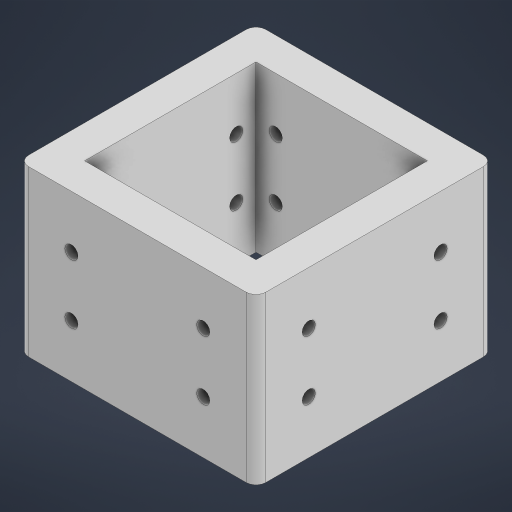
# Autodesk Inventor part: centerlegg_mounting_bracket
Saved by Autodesk Inventor 2024 (Build 280153000, 153)
## iProperties
Created: 2023-05-23
Part Number: centerlegg_mounting_bracket
Material: Generic
Document SubType Name: Modeling
Designer: aasmu
Density: 1 g/cm^3
Appearance: Default
screw_size: 4.000 mm
boarder_to_hole: 16.000 mm
bracket_height: 50.000 mm
Author: aasmu
Autodesk Inventor part; units mm, degrees
ref_plane "YZ Plane" through (0, 0, 0) normal (1, 0, 0) x (0, 1, 0)
ref_plane "XZ Plane" through (0, 0, 0) normal (0, 1, 0) x (-1, 0, 0)
ref_plane "XY Plane" through (0, 0, 0) normal (0, 0, 1) x (1, 0, 0)
sketch "Sketch1" plane through (0, 0, 0) normal (0, 1, 0) x (-1, 0, 0)
  line L0 (0, 0) -> (72, 0)
  line L1 (72, 0) -> (72, -72)
  line L2 (72, -72) -> (0, -72)
  line L3 (0, -72) -> (0, 0)
  line L4 (62, -10) -> (10, -10)
  line L5 (10, -10) -> (10, -62)
  line L6 (10, -62) -> (62, -62)
  line L7 (62, -62) -> (62, -10)
  line L8 (36, 0) -> (36, -10) construction
  line L9 (10, -36) -> (0, -36) construction
  dimension "d1" = 52
  dimension "d3" = 10
  constraints: 20 end point, 4 midpoint, 4 parallel, 4 perpendicular, 3 horizontal, 1 vertical
  measures "d1" distance of L5.end L6.end
  measures "d3" distance between parallel lines of L7 L1
extrude "Extrusion1" add sketch "Sketch1" along normal blind 50
sketch "Sketch2" plane through (-72, 0, 0) normal (0, 0, 1) x (1, 0, 0)
  line L0 (10, 50) -> (62, 50) construction
  line L1 (16, 50) -> (16, 34) construction
  line L2 (16, 16) -> (16, 0) construction
  line L3 (16, 34) -> (0, 34) construction
  line L4 (0, 0) -> (0, 50) construction
  line L5 (56, 50) -> (56, 34) construction
  line L6 (56, 34) -> (72, 34) construction
  line L7 (72, 0) -> (72, 50) construction
  line L8 (72, 16) -> (56, 16) construction
  line L9 (56, 16) -> (56, 0) construction
  circle A0 centre (16, 34) radius 2
  circle A1 centre (56, 34) radius 2
  circle A2 centre (56, 16) radius 2
  circle A3 centre (16, 16) radius 2
  line L10 (0, 0) -> (72, 0) construction
  dimension "boarder_to_hole" = 16
  dimension "d7" = 4
  constraints: 15 end point, 7 point on line, 6 equal length, 4 centre point, 4 coincident, 3 equal radius, 2 horizontal, 2 perpendicular, 2 vertical, 1 collinear
  measures "boarder_to_hole" distance of L1.end L1.start
  measures "d7" diameter of A0
extrude "Extrusion2" cut sketch "Sketch2" against normal up to surface (72 mm away)
sketch "Sketch3" plane through (0, 0, 0) normal (1, 0, 0) x (0, 0, -1)
  line L0 (0, 50) -> (60.8888, 50) construction
  line L1 (16, 50) -> (16, 34) construction
  line L2 (16, 16) -> (16, 0) construction
  line L3 (16, 34) -> (0, 34) construction
  line L4 (0, 0) -> (0, 50) construction
  line L5 (56, 50) -> (56, 34) construction
  line L6 (56, 34) -> (72, 34) construction
  line L7 (72, 0) -> (72, 49.9084) construction
  line L8 (72, 16) -> (56, 16) construction
  line L9 (56, 16) -> (56, 0) construction
  circle A0 centre (16, 34) radius 2
  circle A1 centre (56, 34) radius 2
  circle A2 centre (56, 16) radius 2
  circle A3 centre (16, 16) radius 2
  line L10 (0, 0) -> (72, 0) construction
  line L11 (0, 50) -> (72, 50) projected
  dimension "d10" = 16
  dimension "d13" = 4
  constraints: 23 end point, 8 point on line, 6 coincident, 6 equal length, 4 centre point, 4 vertical, 3 equal radius, 3 horizontal, 2 perpendicular, 1 collinear
  measures "d10" distance of L1.end L1.start
  measures "d13" diameter of A0
extrude "Extrusion3" cut sketch "Sketch3" against normal up to surface (72 mm away)
fillet "Fillet1" radius 3 4 edges at (0, 25, 0) (-72, 25, 0) (-72, 25, -72) (0, 25, -72)
equation "\"d3\" = square_thickness"
equation "\"d7\" = screw_size"
equation "\"d10\" = boarder_to_hole"
equation "\"d13\" = screw_size"
equation "\"square_thickness\" = 10"
equation "\"screw_size\" = 4"
body "Solid1"
